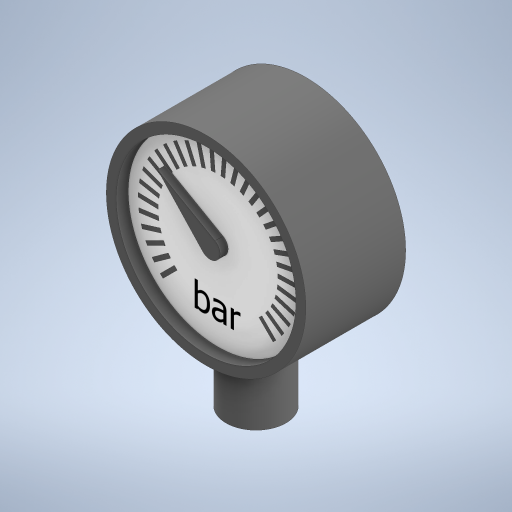
# Autodesk Inventor part: Manometer
Saved by Autodesk Inventor 2023 (Build 270158000, 158)
## iProperties
Created: 2024-12-13
Part Number: Manometer
Material: Generisch
Document SubType Name: Modeling
Designer: aurich
Density: 1 g/cm^3
Appearance: Vorgabe
Author: aurich
Autodesk Inventor part; units mm, degrees
ref_plane "YZ Plane" through (0, 0, 0) normal (1, 0, 0) x (0, 1, 0)
ref_plane "XY Plane" through (0, 0, 0) normal (0, 0, 1) x (1, 0, 0)
sketch "Skizze1" plane through (0, 0, 0) normal (0, 0, 1) x (1, 0, 0)
  circle A0 centre (0, 0) radius 25
  dimension "d0" = 50
  constraints: 1 centre point, 1 coincident
  measures "d0" diameter of A0
extrude "Extrusion1" add sketch "Skizze1" along normal mid plane 25
sketch "Skizze2" plane through (0, 0, 12.5) normal (0, 0, 1) x (1, 0, 0)
  circle A0 centre (0, 0) radius 22.5
  dimension "d3" = 45
  constraints: 1 centre point, 1 coincident
  measures "d3" diameter of A0
extrude "Extrusion2" cut sketch "Skizze2" against normal blind 3
sketch "Skizze3" plane through (0, 0, 9.5) normal (0, 0, 1) x (1, 0, 0)
  line L0 (0, 0) -> (-10.6066, -10.6066) construction
  line L1 (0, 0) -> (21.1652, 0) construction
  circle A0 centre (0, 0) radius 20 construction
  circle A1 centre (0, 0) radius 15 construction
  line L2 (-10.9602, -10.253) -> (-14.4957, -13.7886)
  line L3 (-14.4957, -13.7886) -> (-13.7886, -14.4957)
  line L4 (-13.7886, -14.4957) -> (-10.253, -10.9602)
  line L5 (-10.253, -10.9602) -> (-10.9602, -10.253)
  line L6 (-10.6066, -10.6066) -> (-14.1421, -14.1421) construction
  line L7 (-14.1421, -14.1421) -> (-14.9661, -14.9661) construction
  line L8 (-12.4745, -8.3448) -> (-16.5355, -11.2618)
  line L9 (-16.5355, -11.2618) -> (-15.9521, -12.074)
  line L10 (-15.9521, -12.074) -> (-11.8911, -9.157)
  line L11 (-11.8911, -9.157) -> (-12.4745, -8.3448)
  line L12 (-12.1828, -8.7509) -> (-16.2438, -11.6679) construction
  line L13 (-16.2438, -11.6679) -> (-17.1901, -12.3477) construction
  line L14 (-13.6602, -6.2167) -> (-18.1396, -8.4383)
  line L15 (-18.1396, -8.4383) -> (-17.6953, -9.3342)
  line L16 (-17.6953, -9.3342) -> (-13.2159, -7.1126)
  line L17 (-13.2159, -7.1126) -> (-13.6602, -6.2167)
  line L18 (-13.4381, -6.6647) -> (-17.9174, -8.8862) construction
  line L19 (-17.9174, -8.8862) -> (-18.9613, -9.4039) construction
  line L20 (-14.486, -3.9249) -> (-19.2658, -5.3925)
  line L21 (-19.2658, -5.3925) -> (-18.9723, -6.3484)
  line L22 (-18.9723, -6.3484) -> (-14.1925, -4.8808)
  line L23 (-14.1925, -4.8808) -> (-14.486, -3.9249)
  line L24 (-14.3393, -4.4028) -> (-19.119, -5.8705) construction
  line L25 (-19.119, -5.8705) -> (-20.2329, -6.2125) construction
  line L26 (-14.9302, -1.5296) -> (-19.8844, -2.2046)
  line L27 (-19.8844, -2.2046) -> (-19.7494, -3.1954)
  line L28 (-19.7494, -3.1954) -> (-14.7952, -2.5204)
  line L29 (-14.7952, -2.5204) -> (-14.9302, -1.5296)
  line L30 (-14.8627, -2.025) -> (-19.8169, -2.7) construction
  line L31 (-19.8169, -2.7) -> (-20.9715, -2.8573) construction
  line L32 (-14.981, 0.906) -> (-19.9791, 1.0414)
  line L33 (-19.9791, 1.0414) -> (-20.0062, 0.0418)
  line L34 (-20.0062, 0.0418) -> (-15.008, -0.0936)
  line L35 (-15.008, -0.0936) -> (-14.981, 0.906)
  line L36 (-14.9945, 0.4062) -> (-19.9927, 0.5416) construction
  line L37 (-19.9927, 0.5416) -> (-21.1574, 0.5731) construction
  line L38 (-14.637, 3.3177) -> (-19.5475, 4.2599)
  line L39 (-19.5475, 4.2599) -> (-19.7359, 3.2779)
  line L40 (-19.7359, 3.2779) -> (-14.8255, 2.3356)
  line L41 (-14.8255, 2.3356) -> (-14.637, 3.3177)
  line L42 (-14.7313, 2.8267) -> (-19.6417, 3.7689) construction
  line L43 (-19.6417, 3.7689) -> (-20.786, 3.9885) construction
  line L44 (-13.9075, 5.642) -> (-18.6008, 7.3663)
  line L45 (-18.6008, 7.3663) -> (-18.9456, 6.4276)
  line L46 (-18.9456, 6.4276) -> (-14.2523, 4.7034)
  line L47 (-14.2523, 4.7034) -> (-13.9075, 5.642)
  line L48 (-14.0799, 5.1727) -> (-18.7732, 6.8969) construction
  line L49 (-18.7732, 6.8969) -> (-19.8669, 7.2987) construction
  line L50 (-12.8115, 7.8177) -> (-17.164, 10.2785)
  line L51 (-17.164, 10.2785) -> (-17.6562, 9.408)
  line L52 (-17.6562, 9.408) -> (-13.3036, 6.9472)
  line L53 (-13.3036, 6.9472) -> (-12.8115, 7.8177)
  line L54 (-13.0576, 7.3824) -> (-17.4101, 9.8432) construction
  line L55 (-17.4101, 9.8432) -> (-18.4244, 10.4167) construction
  line L56 (-11.3779, 9.7874) -> (-15.275, 12.9199)
  line L57 (-15.275, 12.9199) -> (-15.9015, 12.1405)
  line L58 (-15.9015, 12.1405) -> (-12.0045, 9.0079)
  line L59 (-12.0045, 9.0079) -> (-11.3779, 9.7874)
  line L60 (-11.6912, 9.3976) -> (-15.5883, 12.5302) construction
  line L61 (-15.5883, 12.5302) -> (-16.4964, 13.2602) construction
  line L62 (-9.6446, 11.4992) -> (-12.9836, 15.2209)
  line L63 (-12.9836, 15.2209) -> (-13.7279, 14.5531)
  line L64 (-13.7279, 14.5531) -> (-10.389, 10.8314)
  line L65 (-10.389, 10.8314) -> (-9.6446, 11.4992)
  line L66 (-10.0168, 11.1653) -> (-13.3558, 14.887) construction
  line L67 (-13.3558, 14.887) -> (-14.1339, 15.7544) construction
  line L68 (-7.6572, 12.908) -> (-10.3501, 17.1209)
  line L69 (-10.3501, 17.1209) -> (-11.1927, 16.5824)
  line L70 (-11.1927, 16.5824) -> (-8.4998, 12.3694)
  line L71 (-8.4998, 12.3694) -> (-7.6572, 12.908)
  line L72 (-8.0785, 12.6387) -> (-10.7714, 16.8516) construction
  line L73 (-10.7714, 16.8516) -> (-11.3989, 17.8334) construction
  line L74 (-5.4681, 13.9768) -> (-7.4439, 18.5698)
  line L75 (-7.4439, 18.5698) -> (-8.3625, 18.1747)
  line L76 (-8.3625, 18.1747) -> (-6.3867, 13.5816)
  line L77 (-6.3867, 13.5816) -> (-5.4681, 13.9768)
  line L78 (-5.9274, 13.7792) -> (-7.9032, 18.3723) construction
  line L79 (-7.9032, 18.3723) -> (-8.3636, 19.4426) construction
  line L80 (-3.1348, 14.6773) -> (-4.3415, 19.5295)
  line L81 (-4.3415, 19.5295) -> (-5.312, 19.2882)
  line L82 (-5.312, 19.2882) -> (-4.1053, 14.4359)
  line L83 (-4.1053, 14.4359) -> (-3.1348, 14.6773)
  line L84 (-3.6201, 14.5566) -> (-4.8268, 19.4088) construction
  line L85 (-4.8268, 19.4088) -> (-5.108, 20.5396) construction
  line L86 (-0.719, 14.9911) -> (-1.1248, 19.9746)
  line L87 (-1.1248, 19.9746) -> (-2.1215, 19.8934)
  line L88 (-2.1215, 19.8934) -> (-1.7157, 14.9099)
  line L89 (-1.7157, 14.9099) -> (-0.719, 14.9911)
  line L90 (-1.2174, 14.9505) -> (-1.6232, 19.934) construction
  line L91 (-1.6232, 19.934) -> (-1.7177, 21.0954) construction
  line L92 (1.7157, 14.9099) -> (2.1215, 19.8934)
  line L93 (2.1215, 19.8934) -> (1.1248, 19.9746)
  line L94 (1.1248, 19.9746) -> (0.719, 14.9911)
  line L95 (0.719, 14.9911) -> (1.7157, 14.9099)
  line L96 (1.2174, 14.9505) -> (1.6232, 19.934) construction
  line L97 (1.6232, 19.934) -> (1.7177, 21.0954) construction
  line L98 (4.1053, 14.4359) -> (5.312, 19.2882)
  line L99 (5.312, 19.2882) -> (4.3415, 19.5295)
  line L100 (4.3415, 19.5295) -> (3.1348, 14.6773)
  line L101 (3.1348, 14.6773) -> (4.1053, 14.4359)
  line L102 (3.6201, 14.5566) -> (4.8268, 19.4088) construction
  line L103 (4.8268, 19.4088) -> (5.108, 20.5396) construction
  line L104 (6.3867, 13.5816) -> (8.3625, 18.1747)
  line L105 (8.3625, 18.1747) -> (7.4439, 18.5698)
  line L106 (7.4439, 18.5698) -> (5.4681, 13.9768)
  line L107 (5.4681, 13.9768) -> (6.3867, 13.5816)
  line L108 (5.9274, 13.7792) -> (7.9032, 18.3723) construction
  line L109 (7.9032, 18.3723) -> (8.3636, 19.4426) construction
  line L110 (8.4998, 12.3694) -> (11.1927, 16.5824)
  line L111 (11.1927, 16.5824) -> (10.3501, 17.1209)
  line L112 (10.3501, 17.1209) -> (7.6572, 12.908)
  line L113 (7.6572, 12.908) -> (8.4998, 12.3694)
  line L114 (8.0785, 12.6387) -> (10.7714, 16.8516) construction
  line L115 (10.7714, 16.8516) -> (11.3989, 17.8334) construction
  line L116 (10.389, 10.8314) -> (13.7279, 14.5531)
  line L117 (13.7279, 14.5531) -> (12.9836, 15.2209)
  line L118 (12.9836, 15.2209) -> (9.6446, 11.4992)
  line L119 (9.6446, 11.4992) -> (10.389, 10.8314)
  line L120 (10.0168, 11.1653) -> (13.3558, 14.887) construction
  line L121 (13.3558, 14.887) -> (14.1339, 15.7544) construction
  line L122 (12.0045, 9.0079) -> (15.9015, 12.1405)
  line L123 (15.9015, 12.1405) -> (15.275, 12.9199)
  line L124 (15.275, 12.9199) -> (11.3779, 9.7874)
  line L125 (11.3779, 9.7874) -> (12.0045, 9.0079)
  line L126 (11.6912, 9.3976) -> (15.5883, 12.5302) construction
  line L127 (15.5883, 12.5302) -> (16.4964, 13.2602) construction
  line L128 (13.3036, 6.9472) -> (17.6562, 9.408)
  line L129 (17.6562, 9.408) -> (17.164, 10.2785)
  line L130 (17.164, 10.2785) -> (12.8115, 7.8177)
  line L131 (12.8115, 7.8177) -> (13.3036, 6.9472)
  line L132 (13.0576, 7.3824) -> (17.4101, 9.8432) construction
  line L133 (17.4101, 9.8432) -> (18.4244, 10.4167) construction
  line L134 (14.2523, 4.7034) -> (18.9456, 6.4276)
  line L135 (18.9456, 6.4276) -> (18.6008, 7.3663)
  line L136 (18.6008, 7.3663) -> (13.9075, 5.642)
  line L137 (13.9075, 5.642) -> (14.2523, 4.7034)
  line L138 (14.0799, 5.1727) -> (18.7732, 6.8969) construction
  line L139 (18.7732, 6.8969) -> (19.8669, 7.2987) construction
  line L140 (14.8255, 2.3356) -> (19.7359, 3.2779)
  line L141 (19.7359, 3.2779) -> (19.5475, 4.2599)
  line L142 (19.5475, 4.2599) -> (14.637, 3.3177)
  line L143 (14.637, 3.3177) -> (14.8255, 2.3356)
  line L144 (14.7313, 2.8267) -> (19.6417, 3.7689) construction
  line L145 (19.6417, 3.7689) -> (20.786, 3.9885) construction
  line L146 (15.008, -0.0936) -> (20.0062, 0.0418)
  line L147 (20.0062, 0.0418) -> (19.9791, 1.0414)
  line L148 (19.9791, 1.0414) -> (14.981, 0.906)
  line L149 (14.981, 0.906) -> (15.008, -0.0936)
  line L150 (14.9945, 0.4062) -> (19.9927, 0.5416) construction
  line L151 (19.9927, 0.5416) -> (21.1574, 0.5731) construction
  line L152 (14.7952, -2.5204) -> (19.7494, -3.1954)
  line L153 (19.7494, -3.1954) -> (19.8844, -2.2046)
  line L154 (19.8844, -2.2046) -> (14.9302, -1.5296)
  line L155 (14.9302, -1.5296) -> (14.7952, -2.5204)
  line L156 (14.8627, -2.025) -> (19.8169, -2.7) construction
  line L157 (19.8169, -2.7) -> (20.9715, -2.8573) construction
  line L158 (14.1925, -4.8808) -> (18.9723, -6.3484)
  line L159 (18.9723, -6.3484) -> (19.2658, -5.3925)
  line L160 (19.2658, -5.3925) -> (14.486, -3.9249)
  line L161 (14.486, -3.9249) -> (14.1925, -4.8808)
  line L162 (14.3393, -4.4028) -> (19.119, -5.8705) construction
  line L163 (19.119, -5.8705) -> (20.2329, -6.2125) construction
  line L164 (13.2159, -7.1126) -> (17.6953, -9.3342)
  line L165 (17.6953, -9.3342) -> (18.1396, -8.4383)
  line L166 (18.1396, -8.4383) -> (13.6602, -6.2167)
  line L167 (13.6602, -6.2167) -> (13.2159, -7.1126)
  line L168 (13.4381, -6.6647) -> (17.9174, -8.8862) construction
  line L169 (17.9174, -8.8862) -> (18.9613, -9.4039) construction
  line L170 (11.8911, -9.157) -> (15.9521, -12.074)
  line L171 (15.9521, -12.074) -> (16.5355, -11.2618)
  line L172 (16.5355, -11.2618) -> (12.4745, -8.3448)
  line L173 (12.4745, -8.3448) -> (11.8911, -9.157)
  line L174 (12.1828, -8.7509) -> (16.2438, -11.6679) construction
  line L175 (16.2438, -11.6679) -> (17.1901, -12.3477) construction
  line L176 (10.253, -10.9602) -> (13.7886, -14.4957)
  line L177 (13.7886, -14.4957) -> (14.4957, -13.7886)
  line L178 (14.4957, -13.7886) -> (10.9602, -10.253)
  line L179 (10.9602, -10.253) -> (10.253, -10.9602)
  line L180 (10.6066, -10.6066) -> (14.1421, -14.1421) construction
  line L181 (14.1421, -14.1421) -> (14.9661, -14.9661) construction
  dimension "d7" = 40
  dimension "d8" = 30
  dimension "d6" = 135
  dimension "d9" = 0.5
  dimension "d10" = 0.5
  dimension "d13" = 270
  constraints: 364 end point, 60 midpoint, 5 perpendicular, 3 parallel, 2 coincident, 1 horizontal, 384 other
  measures "d6" angle of L0 L1
  measures "d9" distance between parallel lines of L0 L2
  measures "d10" distance between parallel lines of L4 L0
extrude "Extrusion3" add sketch "Skizze3" along normal blind 0.01
sketch "Skizze4" plane through (0, 0, 9.5) normal (0, 0, 1) x (1, 0, 0)
  arc A0 (-1.8249, -1.7088) -> (1.2397, 2.171) centre (0, 0) ccw
  line L0 (-13.1537, 10.3898) -> (-1.8249, -1.7088)
  line L1 (-13.1537, 10.3898) -> (1.2397, 2.171)
  line L2 (0, 0) -> (-19.6182, 15.496) construction
  circle A1 centre (0, 0) radius 25 projected
  dimension "d17" = 5
  constraints: 6 end point, 2 point on circle, 2 tangent, 1 centre point, 1 coincident, 1 point on line, 2 other
  measures "d17" diameter of A0
extrude "Extrusion4" add sketch "Skizze4" along normal blind 2 contours L0 L1 A0
ref_plane "Arbeitsebene1" through (0, -25, 0) normal (0, 1, 0) x (-1, 0, 0)
sketch "Skizze5" plane through (0, -25, 0) normal (0, 1, 0) x (-1, 0, 0)
  circle A0 centre (0, 0) radius 7.5
  dimension "d20" = 15
  constraints: 1 centre point, 1 coincident
  measures "d20" diameter of A0
extrude "Extrusion5" add sketch "Skizze5" along normal mid plane 30
sketch "Skizze6" plane through (0, 0, 9.5) normal (0, 0, 1) x (1, 0, 0)
  line L0 (-6.4147, -10.5001) -> (5.6518, -10.5001) construction
  line L1 (5.6518, -10.5001) -> (5.6518, -17.0005) construction
  line L2 (5.6518, -17.0005) -> (-6.4147, -17.0005) construction
  line L3 (-6.4147, -17.0005) -> (-6.4147, -10.5001) construction
  point P0 (0, 0)
  constraints: 2 other
